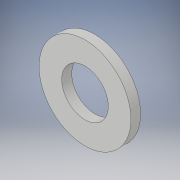
# Autodesk Inventor part: lavirinthos_exodos
Saved by Autodesk Inventor 2019 (Build 230136000, 136)
## iProperties
Created: 2021-01-02
Part Number: lavirinthos_exodos
Material: Generic
Document SubType Name: Modeling
Designer: Dimitris
Density: 1 g/cm^3
Appearance: Default
Author: Dimitris
Autodesk Inventor part; units mm, degrees
ref_plane "YZ Plane" through (0, 0, 0) normal (1, 0, 0) x (0, 1, 0)
ref_plane "XZ Plane" through (0, 0, 0) normal (0, 1, 0) x (-1, 0, 0)
ref_plane "XY Plane" through (0, 0, 0) normal (0, 0, 1) x (1, 0, 0)
sketch "Sketch2" plane through (0, 0, 0) normal (0, 0, 1) x (1, 0, 0)
  circle A0 centre (0, 0) radius 70
  circle A1 centre (0, 0) radius 138
  dimension "d1" = 140
  dimension "d2" = 276
  constraints: 2 centre point, 2 coincident
  measures "d1" diameter of A0
  measures "d2" diameter of A1
extrude "Extrusion1" add sketch "Sketch2" along normal blind 30
sketch "Sketch5" plane through (0, 0, 0) normal (1, 0, 0) x (0, 1, 0)
  line L0 (-138, 0) -> (138, 0) projected
  line L1 (72.7156, 0) -> (114.2156, 0)
  line L2 (114.2156, 0) -> (114.2156, 11)
  line L3 (114.2156, 11) -> (119.2156, 11)
  line L4 (119.2156, 11) -> (119.2156, 1)
  line L5 (119.2156, 1) -> (122.2156, 1)
  line L6 (122.2156, 1) -> (122.2156, 11)
  line L7 (122.2156, 11) -> (127.2156, 11)
  line L8 (127.2156, 11) -> (127.2156, 1)
  line L9 (127.2156, 1) -> (130.2156, 1)
  line L10 (130.2156, 1) -> (130.2156, 11)
  line L11 (130.2156, 11) -> (135.2156, 11)
  line L12 (135.2156, 11) -> (135.2156, 1)
  line L13 (135.2156, 1) -> (138, 1)
  line L14 (138, 0) -> (138, 30) projected
  line L15 (0, -6) -> (0, 36) projected
  point P0 (0, 0)
  dimension "d31" = 41.5
  dimension "d32" = 11
  dimension "d33" = 23.7844
  dimension "d34" = 5
  dimension "d35" = 10
  dimension "d36" = 3
  dimension "d37" = 10
  dimension "d38" = 5
  dimension "d39" = 10
  dimension "d40" = 3
  dimension "d41" = 10
  dimension "d42" = 5
  dimension "d43" = 10
  constraints: 26 end point, 6 perpendicular, 3 horizontal, 3 point on line, 2 vertical, 1 parallel
  measures "d31" distance of L1.start L1.end
  measures "d32" distance of L1.end L2.end
  measures "d33" distance from line of L0.end L2
  measures "d34" distance of L2.end L3.end
  measures "d35" distance of L3.end L4.end
  measures "d36" distance of L4.end L5.end
  measures "d37" distance of L5.end L6.end
  measures "d38" distance of L6.end L7.end
  measures "d39" distance of L7.end L8.end
  measures "d40" distance of L8.end L9.end
  measures "d41" distance of L9.end L10.end
  measures "d42" distance of L10.end L11.end
  measures "d43" distance of L11.end L12.end
revolve "Revolution3" cut sketch "Sketch5" angle 360 about axis through (0, 0, -10) along (0, 0, 1)
body "Solid1"
